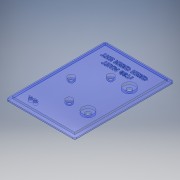
# Autodesk Inventor part: top
Saved by Autodesk Inventor 2017 SP1 (Build 210196100, 196)
## iProperties
Created: 2016-12-24
Part Number: top
Material: Generic
Document SubType Name: Modeling
Designer: wsh32
Density: 1 g/cm^3
Appearance: Clear - Blue
Author: wsh32
Autodesk Inventor part; units mm, degrees
ref_plane "YZ Plane" through (0, 0, 0) normal (1, 0, 0) x (0, 1, 0)
ref_plane "XZ Plane" through (0, 0, 0) normal (0, 1, 0) x (-1, 0, 0)
ref_plane "XY Plane" through (0, 0, 0) normal (0, 0, 1) x (1, 0, 0)
sketch "Sketch1" plane through (0, 0, 0) normal (0, 1, 0) x (-1, 0, 0)
  line L0 (0, 0) -> (-106.68, 0)
  line L1 (-106.68, 0) -> (-106.68, -153.67)
  line L2 (-106.68, -153.67) -> (0, -153.67)
  line L3 (0, -153.67) -> (0, 0)
  dimension "d0" = 153.67
  dimension "d1" = 106.68
  constraints: 8 end point, 2 parallel, 1 horizontal, 1 perpendicular
  measures "d0" distance of L2.end L0.start
  measures "d1" distance of L1.end L2.end
extrude "Extrusion1" add sketch "Sketch1" along normal blind 3.175
sketch "Sketch2" plane through (0, 3.175, 0) normal (0, 1, 0) x (1, 0, 0)
  line L0 (0, 0) -> (106.68, 0) projected
  line L1 (106.68, 0) -> (106.68, 153.67) projected
  line L2 (106.68, 153.67) -> (0, 153.67) projected
  line L3 (0, 153.67) -> (0, 0) projected
  line L4 (5.08, 5.08) -> (101.6, 5.08)
  line L5 (101.6, 5.08) -> (101.6, 148.59)
  line L6 (101.6, 148.59) -> (5.08, 148.59)
  line L7 (5.08, 148.59) -> (5.08, 5.08)
  dimension "d4" = 5.08
  constraints: 8 end point, 3 other
  measures "d4" distance between parallel lines of L3 L7
extrude "Extrusion2" add sketch "Sketch2" along normal blind 3.175 contours L7 L6 L5 L4
chamfer "Chamfer1" distance 1.27 angle 45 4 edges at (53.34, 0, 0) (0, 0, -76.835) (106.68, 0, -76.835) (53.34, 0, -153.67)
fillet "Fillet1" radius 3.175 4 edges at (0, 2.2225, -153.67) (0, 2.2225, 0) (106.68, 2.2225, 0) (106.68, 2.2225, -153.67)
sketch "Sketch6" plane through (0, 6.35, 0) normal (0, 1, 0) x (1, 0, 0)
  line L0 (5.08, 5.08) -> (101.6, 5.08) construction
  line L1 (101.6, 5.08) -> (101.6, 148.59) construction
  line L2 (101.6, 148.59) -> (5.08, 148.59) construction
  line L3 (5.08, 148.59) -> (5.08, 5.08) construction
  line L4 (53.34, 108.9244) -> (82.296, 108.9244) construction
  line L5 (82.296, 108.9244) -> (82.296, 44.7456) construction
  line L6 (82.296, 44.7456) -> (53.34, 44.7456) construction
  line L7 (53.34, 44.7456) -> (53.34, 108.9244) construction
  line L8 (53.34, 76.835) -> (82.296, 76.835) construction
  point P0 (0, 0)
  point P1 (24.384, 76.835)
  dimension "d39" = 39.6656
  dimension "d40" = 39.6656
  dimension "d41" = 64.1789
  dimension "d42" = 19.304
  dimension "d43" = 19.304
  dimension "d44" = 57.912
  dimension "d45" = 28.956
  dimension "d46" = 28.956
  constraints: 10 end point, 3 coincident, 2 midpoint, 2 parallel, 1 horizontal, 1 perpendicular, 1 point on line
  measures "d39" distance between parallel lines of L2 L4
  measures "d40" distance between parallel lines of L0 L6
  measures "d41" distance between parallel lines of L6 L4
  measures "d42" distance from line of L3 point (24.384, 76.835)
  measures "d43" distance between parallel lines of L1 L5
  measures "d44" distance from line of L5 point (24.384, 76.835)
  measures "d45" distance from line of point (24.384, 76.835) L7
  measures "d46" distance between parallel lines of L5 L7
hole "Hole3" at (53.34, 6.35, -108.9244) at (53.34, 6.35, -44.7456) at (24.384, 6.35, -76.835) direction (0, -1, 0) diameter 6.35 end through all counterbore diameter 10.16 counterbore depth 4.1275
sketch "Sketch7" plane through (0, 6.35, 0) normal (0, 1, 0) x (1, 0, 0)
  circle A0 centre (24.384, 76.835) radius 3.175 construction
  circle A1 centre (53.34, 108.9244) radius 3.175 construction
  circle A2 centre (53.34, 44.7456) radius 3.175 construction
  circle A3 centre (53.34, 108.9244) radius 3.175 construction
  line L0 (53.34, 108.9244) -> (82.296, 108.9244) construction
  line L1 (82.296, 108.9244) -> (82.296, 44.7456) construction
  line L2 (82.296, 44.7456) -> (53.34, 44.7456) construction
  line L3 (53.34, 44.7456) -> (53.34, 108.9244) construction
  point P0 (0, 0)
  dimension "d54" = 28.956
  dimension "d55" = 28.956
  constraints: 8 end point, 3 coincident, 2 parallel, 1 horizontal, 1 perpendicular
  measures "d54" distance from line of A0.centre L3
  measures "d55" distance between parallel lines of L1 L3
hole "Hole4" at (82.296, 6.35, -108.9244) at (82.296, 6.35, -44.7456) direction (0, -1, 0) diameter 7.62 end through all counterbore diameter 17.78 counterbore depth 3.81
sketch "Sketch8" plane through (0, 0, 0) normal (0, -1, 0) x (1, 0, 0)
  circle A0 centre (26.67, -19.05) radius 2.921
  circle A1 centre (19.05, -19.05) radius 2.921
  line L0 (26.67, -19.05) -> (19.05, -19.05) construction
  line L1 (0, -3.175) -> (0, -150.495) construction
  line L2 (103.505, 0) -> (3.175, 0) construction
  point P0 (0, 0)
  dimension "d63" = 5.842
  dimension "d64" = 7.62
  dimension "d65" = 19.05
  dimension "d66" = 19.05
  constraints: 2 centre point, 2 end point, 1 equal radius, 1 horizontal
  measures "d63" diameter of A1
  measures "d64" distance of L0.start L0.end
  measures "d65" distance from line of L1 L0.end
  measures "d66" distance between parallel lines of L2 L0
extrude "Extrusion4" cut sketch "Sketch8" against normal blind 3.175
sketch "Sketch9" plane through (26.67, 3.175, -19.05) normal (0, -1, 0) x (1, 0, 0)
  line L0 (0, 0) -> (-7.62, 0) construction
  circle A0 centre (0, 0) radius 2.921 construction
  circle A1 centre (-7.62, 0) radius 2.921 construction
  circle A2 centre (55.626, -89.8744) radius 3.81 construction
  circle A3 centre (55.626, -25.6956) radius 3.81 construction
  circle A4 centre (26.67, -25.6956) radius 3.175 construction
  circle A5 centre (26.67, -89.8744) radius 3.175 construction
  circle A6 centre (-2.286, -57.785) radius 3.175 construction
  line L1 (-25.4, 17.78) -> (78.74, 17.78) construction
  line L2 (-25.4, -133.35) -> (-25.4, 17.78) construction
  line L3 (78.74, -133.35) -> (-25.4, -133.35) construction
  line L4 (78.74, 17.78) -> (78.74, -133.35) construction
  point P0 (-26.67, 19.05)
  point P1 (1.5875, 0)
  point P2 (-1.5875, 0)
  point P3 (-6.0325, 0)
  point P4 (-9.2075, 0)
  dimension "d69" = 1.5875
  dimension "d70" = 1.5875
  dimension "d71" = 1.5875
  dimension "d72" = 1.5875
  dimension "d73" = 3.175
  constraints: 4 point on line, 2 coincident, 2 end point, 1 horizontal
  measures "d69" distance of L0.start point (1.587, 0)
  measures "d70" distance of L0.start point (-1.587, 0)
  measures "d71" distance of L0.end point (-6.032, 0)
  measures "d72" distance of L0.end point (-9.207, 0)
  measures "d73" distance of point (-1.587, 0) point (1.587, 0)
hole "Hole5" at (28.2575, 3.175, -19.05) at (25.0825, 3.175, -19.05) at (20.6375, 3.175, -19.05) at (17.4625, 3.175, -19.05) direction (0, 1, 0) diameter 2.032 end through all
sketch "Sketch10" plane through (0, 0, 0) normal (0, -1, 0) x (1, 0, 0)
  line L0 (8.89, -119.38) -> (85.09, -119.38) construction
  line L1 (85.09, -119.38) -> (85.09, -144.78) construction
  line L2 (85.09, -144.78) -> (8.89, -144.78) construction
  line L3 (8.89, -144.78) -> (8.89, -119.38) construction
  line L4 (5.08, -148.59) -> (5.08, -5.08) projected
  line L5 (5.08, -148.59) -> (101.6, -148.59) projected
  line L6 (25.0464, -130.1787) -> (25.0464, -125.2436)
  line L7 (25.0464, -125.2436) -> (23.2433, -125.2436)
  line L8 (23.2433, -125.2436) -> (23.2433, -124.0827)
  line L9 (23.2433, -124.0827) -> (28.3809, -124.0827)
  line L10 (28.3809, -124.0827) -> (28.3809, -125.2436)
  line L11 (28.3809, -125.2436) -> (26.5778, -125.2436)
  line L12 (26.5778, -125.2436) -> (26.5778, -130.1787)
  line L13 (26.5778, -130.1787) -> (25.0464, -130.1787)
  line L14 (29.0083, -130.1787) -> (29.0083, -124.0827)
  line L15 (29.0083, -124.0827) -> (33.1283, -124.0827)
  line L16 (33.1283, -124.0827) -> (33.1283, -125.2436)
  line L17 (33.1283, -125.2436) -> (30.5298, -125.2436)
  line L18 (30.5298, -125.2436) -> (30.5298, -126.3156)
  line L19 (30.5298, -126.3156) -> (32.9257, -126.3156)
  line L20 (32.9257, -126.3156) -> (32.9257, -127.4765)
  line L21 (32.9257, -127.4765) -> (30.5298, -127.4765)
  line L22 (30.5298, -127.4765) -> (30.5298, -129.0178)
  line L23 (30.5298, -129.0178) -> (33.1283, -129.0178)
  line L24 (33.1283, -129.0178) -> (33.1283, -130.1787)
  line L25 (33.1283, -130.1787) -> (29.0083, -130.1787)
  line L26 (33.5087, -130.1787) -> (35.5686, -124.0827)
  line L27 (35.5686, -124.0827) -> (37.2384, -124.0827)
  line L28 (37.2384, -124.0827) -> (39.2984, -130.1787)
  line L29 (39.2984, -130.1787) -> (37.7225, -130.1787)
  line L30 (37.7225, -130.1787) -> (37.3421, -128.9338)
  line L31 (37.3421, -128.9338) -> (35.4254, -128.9338)
  line L32 (35.4254, -128.9338) -> (35.0401, -130.1787)
  line L33 (35.0401, -130.1787) -> (33.5087, -130.1787)
  line L34 (37.0062, -127.8273) -> (36.3838, -125.8117)
  line L35 (36.3838, -125.8117) -> (35.7564, -127.8273)
  line L36 (35.7564, -127.8273) -> (37.0062, -127.8273)
  line L37 (46.1304, -130.1787) -> (44.6089, -130.1787)
  line L38 (44.6089, -130.1787) -> (44.6089, -126.1378)
  line L39 (44.6089, -126.1378) -> (43.5023, -128.7461)
  line L40 (43.5023, -128.7461) -> (42.4551, -128.7461)
  line L41 (42.4551, -128.7461) -> (41.3485, -126.1378)
  line L42 (41.3485, -126.1378) -> (41.3485, -130.1787)
  line L43 (41.3485, -130.1787) -> (39.906, -130.1787)
  line L44 (39.906, -130.1787) -> (39.906, -124.0827)
  line L45 (39.906, -124.0827) -> (41.6696, -124.0827)
  line L46 (41.6696, -124.0827) -> (43.0232, -127.0912)
  line L47 (43.0232, -127.0912) -> (44.3668, -124.0827)
  line L48 (44.3668, -124.0827) -> (46.1304, -124.0827)
  line L49 (46.1304, -124.0827) -> (46.1304, -130.1787)
  spline S0 degree 2 poles (54.2815, -128.1039) (54.2815, -129.0672) (53.0613, -130.3071) (51.9943, -130.3071) knots 0 0 0 1 2 2 2
  spline S1 degree 2 poles (51.9943, -130.3071) (51.4607, -130.3071) (50.6259, -130.0009) (50.3344, -129.6995) knots 0 0 0 1 2 2 2
  spline S2 degree 2 poles (50.3344, -129.6995) (49.9886, -129.3488) (49.6181, -128.2373) (49.6181, -127.4617) knots 0 0 0 1 2 2 2
  spline S3 degree 2 poles (49.6181, -127.4617) (49.6181, -126.6614) (49.9639, -125.4165) (50.3542, -124.9373) knots 0 0 0 1 2 2 2
  spline S4 degree 2 poles (50.3542, -124.9373) (50.7247, -124.4829) (51.93, -123.9691) (52.755, -123.9691) knots 0 0 0 1 2 2 2
  spline S5 degree 2 poles (52.755, -123.9691) (53.0564, -123.9691) (53.659, -124.0481) (53.7677, -124.0728) knots 0 0 0 1 2 2 2
  line L50 (53.7677, -124.0728) -> (53.7677, -125.2683)
  line L51 (53.7677, -125.2683) -> (53.659, -125.2683)
  spline S6 degree 2 poles (53.659, -125.2683) (53.5504, -125.214) (53.0564, -125.0806) (52.7402, -125.0806) knots 0 0 0 1 2 2 2
  spline S7 degree 2 poles (52.7402, -125.0806) (52.0239, -125.0806) (51.2434, -125.8364) (51.1495, -126.5379) knots 0 0 0 1 2 2 2
  spline S8 degree 2 poles (51.1495, -126.5379) (51.4508, -126.3452) (52.0684, -126.118) (52.4586, -126.118) knots 0 0 0 1 2 2 2
  spline S9 degree 2 poles (52.4586, -126.118) (52.7896, -126.118) (53.3676, -126.2958) (53.5899, -126.4638) knots 0 0 0 1 2 2 2
  spline S10 degree 2 poles (53.5899, -126.4638) (53.906, -126.7059) (54.2815, -127.4913) (54.2815, -128.1039) knots 0 0 0 1 2 2 2
  spline S11 degree 2 poles (52.4981, -129.0227) (52.6167, -128.8745) (52.7451, -128.5287) (52.7451, -128.178) knots 0 0 0 1 2 2 2
  spline S12 degree 2 poles (52.7451, -128.178) (52.7451, -127.8816) (52.5969, -127.4963) (52.4636, -127.3827) knots 0 0 0 1 2 2 2
  spline S13 degree 2 poles (52.4636, -127.3827) (52.3252, -127.2641) (51.9844, -127.1801) (51.7917, -127.1801) knots 0 0 0 1 2 2 2
  spline S14 degree 2 poles (51.7917, -127.1801) (51.6287, -127.1801) (51.2928, -127.2641) (51.1446, -127.3234) knots 0 0 0 1 2 2 2
  spline S15 degree 2 poles (51.1446, -127.3234) (51.1446, -127.3629) (51.1347, -127.5506) (51.1347, -127.6939) knots 0 0 0 1 2 2 2
  spline S16 degree 2 poles (51.1347, -127.6939) (51.1347, -128.2225) (51.3175, -128.8597) (51.4607, -129.0227) knots 0 0 0 1 2 2 2
  spline S17 degree 2 poles (51.4607, -129.0227) (51.5645, -129.1561) (51.8411, -129.2697) (51.9893, -129.2697) knots 0 0 0 1 2 2 2
  spline S18 degree 2 poles (51.9893, -129.2697) (52.1128, -129.2697) (52.3993, -129.1462) (52.4981, -129.0227) knots 0 0 0 1 2 2 2
  spline S19 degree 2 poles (59.6414, -128.4843) (59.6414, -128.8745) (59.3154, -129.5513) (59.0042, -129.7983) knots 0 0 0 1 2 2 2
  spline S20 degree 2 poles (59.0042, -129.7983) (58.6929, -130.0453) (57.7988, -130.322) (57.2208, -130.322) knots 0 0 0 1 2 2 2
  spline S21 degree 2 poles (57.2208, -130.322) (56.6033, -130.322) (55.6795, -130.0404) (55.3831, -129.7983) knots 0 0 0 1 2 2 2
  spline S22 degree 2 poles (55.3831, -129.7983) (55.0917, -129.5563) (54.815, -128.8992) (54.815, -128.5337) knots 0 0 0 1 2 2 2
  spline S23 degree 2 poles (54.815, -128.5337) (54.815, -128.01) (55.393, -127.3135) (55.9413, -127.0813) knots 0 0 0 1 2 2 2
  line L52 (55.9413, -127.0813) -> (55.9413, -127.0566)
  spline S24 degree 2 poles (55.9413, -127.0566) (55.4029, -126.7948) (54.978, -126.0488) (54.978, -125.5894) knots 0 0 0 1 2 2 2
  spline S25 degree 2 poles (54.978, -125.5894) (54.978, -125.2535) (55.2744, -124.6656) (55.5659, -124.4335) knots 0 0 0 1 2 2 2
  spline S26 degree 2 poles (55.5659, -124.4335) (55.8475, -124.2111) (56.7021, -123.9444) (57.2356, -123.9444) knots 0 0 0 1 2 2 2
  spline S27 degree 2 poles (57.2356, -123.9444) (57.7988, -123.9444) (58.6386, -124.1864) (58.9103, -124.3841) knots 0 0 0 1 2 2 2
  spline S28 degree 2 poles (58.9103, -124.3841) (59.1869, -124.5817) (59.4833, -125.1547) (59.4833, -125.4857) knots 0 0 0 1 2 2 2
  spline S29 degree 2 poles (59.4833, -125.4857) (59.4833, -125.9204) (58.9795, -126.6169) (58.4608, -126.859) knots 0 0 0 1 2 2 2
  line L53 (58.4608, -126.859) -> (58.4608, -126.8788)
  spline S30 degree 2 poles (58.4608, -126.8788) (59.0684, -127.1258) (59.6414, -127.9261) (59.6414, -128.4843) knots 0 0 0 1 2 2 2
  spline S31 degree 2 poles (58.1298, -128.5485) (58.1298, -128.2472) (57.8729, -127.931) (57.4579, -127.7285) knots 0 0 0 1 2 2 2
  spline S32 degree 2 poles (57.4579, -127.7285) (57.3394, -127.6741) (56.8898, -127.5012) (56.7169, -127.4271) knots 0 0 0 1 2 2 2
  spline S33 degree 2 poles (56.7169, -127.4271) (56.5588, -127.5852) (56.3069, -128.0594) (56.3069, -128.341) knots 0 0 0 1 2 2 2
  spline S34 degree 2 poles (56.3069, -128.341) (56.3069, -128.7659) (56.8503, -129.2747) (57.29, -129.2747) knots 0 0 0 1 2 2 2
  spline S35 degree 2 poles (57.29, -129.2747) (57.4135, -129.2747) (57.7198, -129.1956) (57.8383, -129.1166) knots 0 0 0 1 2 2 2
  spline S36 degree 2 poles (57.8383, -129.1166) (57.9717, -129.0227) (58.1298, -128.7659) (58.1298, -128.5485) knots 0 0 0 1 2 2 2
  spline S37 degree 2 poles (57.9964, -125.6635) (57.9964, -125.3523) (57.5864, -124.9818) (57.2356, -124.9818) knots 0 0 0 1 2 2 2
  spline S38 degree 2 poles (57.2356, -124.9818) (56.8997, -124.9818) (56.4897, -125.3177) (56.4897, -125.5647) knots 0 0 0 1 2 2 2
  spline S39 degree 2 poles (56.4897, -125.5647) (56.4897, -125.8068) (56.7367, -126.1081) (56.9985, -126.2316) knots 0 0 0 1 2 2 2
  spline S40 degree 2 poles (56.9985, -126.2316) (57.1121, -126.2909) (57.4283, -126.4144) (57.6901, -126.5132) knots 0 0 0 1 2 2 2
  spline S41 degree 2 poles (57.6901, -126.5132) (57.8482, -126.3057) (57.9964, -125.9155) (57.9964, -125.6635) knots 0 0 0 1 2 2 2
  line L54 (64.863, -125.293) -> (62.2596, -130.1787)
  line L55 (62.2596, -130.1787) -> (60.5603, -130.1787)
  line L56 (60.5603, -130.1787) -> (63.2822, -125.2337)
  line L57 (63.2822, -125.2337) -> (60.3775, -125.2337)
  line L58 (60.3775, -125.2337) -> (60.3775, -124.0827)
  line L59 (60.3775, -124.0827) -> (64.863, -124.0827)
  line L60 (64.863, -124.0827) -> (64.863, -125.293)
  line L61 (67.4862, -130.1787) -> (66.0388, -130.1787)
  line L62 (66.0388, -130.1787) -> (66.0388, -128.5683)
  line L63 (66.0388, -128.5683) -> (67.4862, -128.5683)
  line L64 (67.4862, -128.5683) -> (67.4862, -130.1787)
  line L65 (67.4862, -127.19) -> (66.0388, -127.19)
  line L66 (66.0388, -127.19) -> (66.0388, -125.5795)
  line L67 (66.0388, -125.5795) -> (67.4862, -125.5795)
  line L68 (67.4862, -125.5795) -> (67.4862, -127.19)
  line L69 (13.9634, -140.2156) -> (13.9634, -135.2805)
  line L70 (13.9634, -135.2805) -> (12.1603, -135.2805)
  line L71 (12.1603, -135.2805) -> (12.1603, -134.1196)
  line L72 (12.1603, -134.1196) -> (17.2979, -134.1196)
  line L73 (17.2979, -134.1196) -> (17.2979, -135.2805)
  line L74 (17.2979, -135.2805) -> (15.4948, -135.2805)
  line L75 (15.4948, -135.2805) -> (15.4948, -140.2156)
  line L76 (15.4948, -140.2156) -> (13.9634, -140.2156)
  line L77 (23.0679, -140.2156) -> (21.5365, -140.2156)
  line L78 (21.5365, -140.2156) -> (21.5365, -137.5134)
  line L79 (21.5365, -137.5134) -> (19.4567, -137.5134)
  line L80 (19.4567, -137.5134) -> (19.4567, -140.2156)
  line L81 (19.4567, -140.2156) -> (17.9253, -140.2156)
  line L82 (17.9253, -140.2156) -> (17.9253, -134.1196)
  line L83 (17.9253, -134.1196) -> (19.4567, -134.1196)
  line L84 (19.4567, -134.1196) -> (19.4567, -136.3525)
  line L85 (19.4567, -136.3525) -> (21.5365, -136.3525)
  line L86 (21.5365, -136.3525) -> (21.5365, -134.1196)
  line L87 (21.5365, -134.1196) -> (23.0679, -134.1196)
  line L88 (23.0679, -134.1196) -> (23.0679, -140.2156)
  line L89 (24.3325, -140.2156) -> (24.3325, -134.1196)
  line L90 (24.3325, -134.1196) -> (28.4525, -134.1196)
  line L91 (28.4525, -134.1196) -> (28.4525, -135.2805)
  line L92 (28.4525, -135.2805) -> (25.8541, -135.2805)
  line L93 (25.8541, -135.2805) -> (25.8541, -136.3525)
  line L94 (25.8541, -136.3525) -> (28.25, -136.3525)
  line L95 (28.25, -136.3525) -> (28.25, -137.5134)
  line L96 (28.25, -137.5134) -> (25.8541, -137.5134)
  line L97 (25.8541, -137.5134) -> (25.8541, -139.0547)
  line L98 (25.8541, -139.0547) -> (28.4525, -139.0547)
  line L99 (28.4525, -139.0547) -> (28.4525, -140.2156)
  line L100 (28.4525, -140.2156) -> (24.3325, -140.2156)
  line L101 (37.1667, -140.2156) -> (35.6946, -140.2156)
  line L102 (35.6946, -140.2156) -> (33.3432, -135.9672)
  line L103 (33.3432, -135.9672) -> (33.3432, -140.2156)
  line L104 (33.3432, -140.2156) -> (31.9451, -140.2156)
  line L105 (31.9451, -140.2156) -> (31.9451, -134.1196)
  line L106 (31.9451, -134.1196) -> (33.8223, -134.1196)
  line L107 (33.8223, -134.1196) -> (35.7687, -137.6122)
  line L108 (35.7687, -137.6122) -> (35.7687, -134.1196)
  line L109 (35.7687, -134.1196) -> (37.1667, -134.1196)
  line L110 (37.1667, -134.1196) -> (37.1667, -140.2156)
  line L111 (38.4067, -140.2156) -> (38.4067, -134.1196)
  line L112 (38.4067, -134.1196) -> (42.5267, -134.1196)
  line L113 (42.5267, -134.1196) -> (42.5267, -135.2805)
  line L114 (42.5267, -135.2805) -> (39.9282, -135.2805)
  line L115 (39.9282, -135.2805) -> (39.9282, -136.3525)
  line L116 (39.9282, -136.3525) -> (42.3241, -136.3525)
  line L117 (42.3241, -136.3525) -> (42.3241, -137.5134)
  line L118 (42.3241, -137.5134) -> (39.9282, -137.5134)
  line L119 (39.9282, -137.5134) -> (39.9282, -139.0547)
  line L120 (39.9282, -139.0547) -> (42.5267, -139.0547)
  line L121 (42.5267, -139.0547) -> (42.5267, -140.2156)
  line L122 (42.5267, -140.2156) -> (38.4067, -140.2156)
  line L123 (49.1957, -140.2156) -> (47.3333, -140.2156)
  line L124 (47.3333, -140.2156) -> (45.6389, -137.9778)
  line L125 (45.6389, -137.9778) -> (45.0856, -137.9778)
  line L126 (45.0856, -137.9778) -> (45.0856, -140.2156)
  line L127 (45.0856, -140.2156) -> (43.5641, -140.2156)
  line L128 (43.5641, -140.2156) -> (43.5641, -134.1196)
  line L129 (43.5641, -134.1196) -> (46.0143, -134.1196)
  spline S42 degree 2 poles (46.0143, -134.1196) (46.5232, -134.1196) (47.2741, -134.2481) (47.5952, -134.4457) knots 0 0 0 1 2 2 2
  spline S43 degree 2 poles (47.5952, -134.4457) (47.9212, -134.6531) (48.3065, -135.3003) (48.3065, -135.7943) knots 0 0 0 1 2 2 2
  spline S44 degree 2 poles (48.3065, -135.7943) (48.3065, -136.4908) (47.6742, -137.3652) (47.1456, -137.6221) knots 0 0 0 1 2 2 2
  line L130 (47.1456, -137.6221) -> (49.1957, -140.2156)
  spline S45 degree 2 poles (46.7356, -135.9869) (46.7356, -135.7548) (46.5577, -135.4238) (46.3552, -135.3349) knots 0 0 0 1 2 2 2
  spline S46 degree 2 poles (46.3552, -135.3349) (46.2119, -135.2756) (45.8612, -135.241) (45.5994, -135.241) knots 0 0 0 1 2 2 2
  line L131 (45.5994, -135.241) -> (45.0856, -135.241)
  line L132 (45.0856, -135.241) -> (45.0856, -136.8811)
  line L133 (45.0856, -136.8811) -> (45.5253, -136.8811)
  spline S47 degree 2 poles (45.5253, -136.8811) (45.8414, -136.8811) (46.291, -136.802) (46.4441, -136.6785) knots 0 0 0 1 2 2 2
  spline S48 degree 2 poles (46.4441, -136.6785) (46.5923, -136.56) (46.7356, -136.2438) (46.7356, -135.9869) knots 0 0 0 1 2 2 2
  spline S49 degree 2 poles (55.0892, -137.1726) (55.0892, -138.0272) (54.3432, -139.3709) (53.7751, -139.7315) knots 0 0 0 1 2 2 2
  spline S50 degree 2 poles (53.7751, -139.7315) (53.3009, -140.0378) (52.1844, -140.2156) (51.5571, -140.2156) knots 0 0 0 1 2 2 2
  line L134 (51.5571, -140.2156) -> (49.6502, -140.2156)
  line L135 (49.6502, -140.2156) -> (49.6502, -134.1196)
  line L136 (49.6502, -134.1196) -> (51.5373, -134.1196)
  spline S51 degree 2 poles (51.5373, -134.1196) (52.1795, -134.1196) (53.3009, -134.2826) (53.7949, -134.5988) knots 0 0 0 1 2 2 2
  spline S52 degree 2 poles (53.7949, -134.5988) (54.3926, -134.9841) (55.0892, -136.2883) (55.0892, -137.1726) knots 0 0 0 1 2 2 2
  spline S53 degree 2 poles (53.5183, -137.1627) (53.5183, -136.56) (53.1033, -135.7004) (52.6784, -135.4584) knots 0 0 0 1 2 2 2
  spline S54 degree 2 poles (52.6784, -135.4584) (52.3672, -135.2904) (51.6855, -135.2558) (51.2113, -135.2558) knots 0 0 0 1 2 2 2
  line L137 (51.2113, -135.2558) -> (51.1816, -135.2558)
  line L138 (51.1816, -135.2558) -> (51.1816, -139.0745)
  line L139 (51.1816, -139.0745) -> (51.2113, -139.0745)
  spline S55 degree 2 poles (51.2113, -139.0745) (51.725, -139.0745) (52.4314, -139.0399) (52.7525, -138.8373) knots 0 0 0 1 2 2 2
  spline S56 degree 2 poles (52.7525, -138.8373) (53.128, -138.6002) (53.5183, -137.7654) (53.5183, -137.1627) knots 0 0 0 1 2 2 2
  line L140 (63.5959, -140.2156) -> (62.0645, -140.2156)
  line L141 (62.0645, -140.2156) -> (62.0645, -137.5134)
  line L142 (62.0645, -137.5134) -> (59.9848, -137.5134)
  line L143 (59.9848, -137.5134) -> (59.9848, -140.2156)
  line L144 (59.9848, -140.2156) -> (58.4533, -140.2156)
  line L145 (58.4533, -140.2156) -> (58.4533, -134.1196)
  line L146 (58.4533, -134.1196) -> (59.9848, -134.1196)
  line L147 (59.9848, -134.1196) -> (59.9848, -136.3525)
  line L148 (59.9848, -136.3525) -> (62.0645, -136.3525)
  line L149 (62.0645, -136.3525) -> (62.0645, -134.1196)
  line L150 (62.0645, -134.1196) -> (63.5959, -134.1196)
  line L151 (63.5959, -134.1196) -> (63.5959, -140.2156)
  line L152 (64.8606, -140.2156) -> (64.8606, -134.1196)
  line L153 (64.8606, -134.1196) -> (68.9806, -134.1196)
  line L154 (68.9806, -134.1196) -> (68.9806, -135.2805)
  line L155 (68.9806, -135.2805) -> (66.3821, -135.2805)
  line L156 (66.3821, -135.2805) -> (66.3821, -136.3525)
  line L157 (66.3821, -136.3525) -> (68.778, -136.3525)
  line L158 (68.778, -136.3525) -> (68.778, -137.5134)
  line L159 (68.778, -137.5134) -> (66.3821, -137.5134)
  line L160 (66.3821, -137.5134) -> (66.3821, -139.0547)
  line L161 (66.3821, -139.0547) -> (68.9806, -139.0547)
  line L162 (68.9806, -139.0547) -> (68.9806, -140.2156)
  line L163 (68.9806, -140.2156) -> (64.8606, -140.2156)
  line L164 (75.6496, -140.2156) -> (73.7872, -140.2156)
  line L165 (73.7872, -140.2156) -> (72.0928, -137.9778)
  line L166 (72.0928, -137.9778) -> (71.5395, -137.9778)
  line L167 (71.5395, -137.9778) -> (71.5395, -140.2156)
  line L168 (71.5395, -140.2156) -> (70.018, -140.2156)
  line L169 (70.018, -140.2156) -> (70.018, -134.1196)
  line L170 (70.018, -134.1196) -> (72.4682, -134.1196)
  spline S57 degree 2 poles (72.4682, -134.1196) (72.977, -134.1196) (73.7279, -134.2481) (74.049, -134.4457) knots 0 0 0 1 2 2 2
  spline S58 degree 2 poles (74.049, -134.4457) (74.3751, -134.6531) (74.7604, -135.3003) (74.7604, -135.7943) knots 0 0 0 1 2 2 2
  spline S59 degree 2 poles (74.7604, -135.7943) (74.7604, -136.4908) (74.1281, -137.3652) (73.5995, -137.6221) knots 0 0 0 1 2 2 2
  line L171 (73.5995, -137.6221) -> (75.6496, -140.2156)
  spline S60 degree 2 poles (73.1895, -135.9869) (73.1895, -135.7548) (73.0116, -135.4238) (72.8091, -135.3349) knots 0 0 0 1 2 2 2
  spline S61 degree 2 poles (72.8091, -135.3349) (72.6658, -135.2756) (72.3151, -135.241) (72.0533, -135.241) knots 0 0 0 1 2 2 2
  line L172 (72.0533, -135.241) -> (71.5395, -135.241)
  line L173 (71.5395, -135.241) -> (71.5395, -136.8811)
  line L174 (71.5395, -136.8811) -> (71.9792, -136.8811)
  spline S62 degree 2 poles (71.9792, -136.8811) (72.2953, -136.8811) (72.7449, -136.802) (72.898, -136.6785) knots 0 0 0 1 2 2 2
  spline S63 degree 2 poles (72.898, -136.6785) (73.0462, -136.56) (73.1895, -136.2438) (73.1895, -135.9869) knots 0 0 0 1 2 2 2
  spline S64 degree 2 poles (81.5431, -137.1726) (81.5431, -138.0272) (80.7971, -139.3709) (80.229, -139.7315) knots 0 0 0 1 2 2 2
  spline S65 degree 2 poles (80.229, -139.7315) (79.7548, -140.0378) (78.6383, -140.2156) (78.0109, -140.2156) knots 0 0 0 1 2 2 2
  line L175 (78.0109, -140.2156) -> (76.1041, -140.2156)
  line L176 (76.1041, -140.2156) -> (76.1041, -134.1196)
  line L177 (76.1041, -134.1196) -> (77.9912, -134.1196)
  spline S66 degree 2 poles (77.9912, -134.1196) (78.6334, -134.1196) (79.7548, -134.2826) (80.2488, -134.5988) knots 0 0 0 1 2 2 2
  spline S67 degree 2 poles (80.2488, -134.5988) (80.8465, -134.9841) (81.5431, -136.2883) (81.5431, -137.1726) knots 0 0 0 1 2 2 2
  spline S68 degree 2 poles (79.9721, -137.1627) (79.9721, -136.56) (79.5572, -135.7004) (79.1323, -135.4584) knots 0 0 0 1 2 2 2
  spline S69 degree 2 poles (79.1323, -135.4584) (78.8211, -135.2904) (78.1394, -135.2558) (77.6651, -135.2558) knots 0 0 0 1 2 2 2
  line L178 (77.6651, -135.2558) -> (77.6355, -135.2558)
  line L179 (77.6355, -135.2558) -> (77.6355, -139.0745)
  line L180 (77.6355, -139.0745) -> (77.6651, -139.0745)
  spline S70 degree 2 poles (77.6651, -139.0745) (78.1789, -139.0745) (78.8853, -139.0399) (79.2064, -138.8373) knots 0 0 0 1 2 2 2
  spline S71 degree 2 poles (79.2064, -138.8373) (79.5819, -138.6002) (79.9721, -137.7654) (79.9721, -137.1627) knots 0 0 0 1 2 2 2
  point P0 (0, 0)
  dimension "d81" = 25.4
  dimension "d82" = 76.2
  dimension "d83" = 3.81
  dimension "d84" = 3.81
  constraints: 1 horizontal, 2 other
  measures "d81" distance of L2.end L0.start
  measures "d82" distance of L1.end L2.end
  measures "d83" distance between parallel lines of L4 L3
  measures "d84" distance between parallel lines of L5 L2
extrude "Extrusion5" cut sketch "Sketch10" against normal blind 1.27
equation "\"d40\" = d39"
equation "\"d41\" = 1.618 * d39"
equation "\"d43\" = d42"
equation "\"d44\" = 3 * d42"
equation "\"d46\" = d45"
equation "\"d55\" = d54"
equation "\"d70\" = d69"
equation "\"d71\" = d69"
equation "\"d72\" = d69"
equation "\"d84\" = d83"
body "Solid1"
